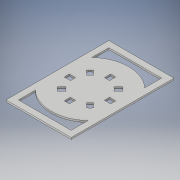
# Autodesk Inventor part: Cuerpo - Base
Saved by Autodesk Inventor 2019 (Build 230136000, 136)
## iProperties
Created: 2020-02-15
Part Number: Cuerpo - Base
Material: Genérico
Document SubType Name: Modeling
Designer: Mafer1
Density: 1 g/cm^3
Appearance: Valor por defecto
Mass: 62.4881 g
Surface Area: 432.904 cm^2
Volume: 62.4881 cm^3
ancho_base: 120.000 mm
largo_base: 200.000 mm
Author: Mafer1
Autodesk Inventor part; units mm, degrees
ref_plane "YZ Plane" through (0, 0, 0) normal (1, 0, 0) x (0, 1, 0)
ref_plane "XZ Plane" through (0, 0, 0) normal (0, 1, 0) x (-1, 0, 0)
ref_plane "XY Plane" through (0, 0, 0) normal (0, 0, 1) x (1, 0, 0)
sketch "Boceto1" plane through (0, 0, 0) normal (0, 1, 0) x (-1, 0, 0)
  line L0 (0, 0) -> (126.6, 0)
  line L1 (126.6, 0) -> (126.6, -200)
  line L2 (126.6, -200) -> (0, -200)
  line L3 (0, -200) -> (0, 0)
  dimension "d0" = 200
  dimension "d1" = 126.6
  constraints: 8 end point, 2 parallel, 1 horizontal, 1 perpendicular
  measures "d0" distance of L0.end L1.end
  measures "d1" distance between parallel lines of L3 L1
extrude "Extrusión1" add sketch "Boceto1" along normal blind 3.3
sketch "Boceto2" plane through (0, 3.3, 0) normal (0, 1, 0) x (1, 0, 0)
  circle A0 centre (-63.3, 100) radius 33.3 construction
  circle A1 centre (-63.3, 100) radius 45.3 construction
  line L0 (-114.6, 155.1217) -> (-114.6, 188)
  line L1 (-114.6, 188) -> (-12, 188)
  line L2 (-12, 188) -> (-12, 155.1217)
  line L3 (-114.6, 44.8783) -> (-114.6, 12)
  line L4 (-114.6, 12) -> (-12, 12)
  line L5 (-12, 12) -> (-12, 44.8783)
  arc A2 (-12, 155.1217) -> (-114.6, 155.1217) centre (-63.3, 100) ccw
  arc A3 (-114.6, 44.8783) -> (-12, 44.8783) centre (-63.3, 100) ccw
  line L6 (-126.6, 0) -> (0, 0) projected
  line L7 (0, 0) -> (0, 200) projected
  line L8 (0, 200) -> (-126.6, 200) projected
  line L9 (-126.6, 200) -> (-126.6, 0) projected
  line L10 (0, 200) -> (-126.6, 200) projected
  line L11 (-68.3, 54.9768) -> (-68.3, 67.0775)
  line L12 (-58.3, 54.9768) -> (-58.3, 67.0775)
  arc A4 (-68.3, 67.0775) -> (-58.3, 67.0775) centre (-63.3, 100) ccw
  arc A5 (-68.3, 54.9768) -> (-58.3, 54.9768) centre (-63.3, 100) ccw
  line L13 (-27.9282, 71.6993) -> (-36.4848, 80.2558)
  arc A6 (-34.9993, 64.6282) -> (-27.9282, 71.6993) centre (-63.3, 100) ccw
  line L14 (-34.9993, 64.6282) -> (-43.5558, 73.1848)
  arc A7 (-43.5558, 73.1848) -> (-36.4848, 80.2558) centre (-63.3, 100) ccw
  line L15 (-18.2768, 105) -> (-30.3775, 105)
  arc A8 (-18.2768, 95) -> (-18.2768, 105) centre (-63.3, 100) ccw
  line L16 (-18.2768, 95) -> (-30.3775, 95)
  arc A9 (-30.3775, 95) -> (-30.3775, 105) centre (-63.3, 100) ccw
  line L17 (-34.9993, 135.3718) -> (-43.5558, 126.8152)
  arc A10 (-27.9282, 128.3007) -> (-34.9993, 135.3718) centre (-63.3, 100) ccw
  line L18 (-27.9282, 128.3007) -> (-36.4848, 119.7442)
  arc A11 (-36.4848, 119.7442) -> (-43.5558, 126.8152) centre (-63.3, 100) ccw
  line L19 (-68.3, 145.0232) -> (-68.3, 132.9225)
  arc A12 (-58.3, 145.0232) -> (-68.3, 145.0232) centre (-63.3, 100) ccw
  line L20 (-58.3, 145.0232) -> (-58.3, 132.9225)
  arc A13 (-58.3, 132.9225) -> (-68.3, 132.9225) centre (-63.3, 100) ccw
  line L21 (-98.6718, 128.3007) -> (-90.1152, 119.7442)
  arc A14 (-91.6007, 135.3718) -> (-98.6718, 128.3007) centre (-63.3, 100) ccw
  line L22 (-91.6007, 135.3718) -> (-83.0442, 126.8152)
  arc A15 (-83.0442, 126.8152) -> (-90.1152, 119.7442) centre (-63.3, 100) ccw
  line L23 (-108.3232, 95) -> (-96.2225, 95)
  arc A16 (-108.3232, 105) -> (-108.3232, 95) centre (-63.3, 100) ccw
  line L24 (-108.3232, 105) -> (-96.2225, 105)
  arc A17 (-96.2225, 105) -> (-96.2225, 95) centre (-63.3, 100) ccw
  line L25 (-91.6007, 64.6282) -> (-83.0442, 73.1848)
  arc A18 (-98.6718, 71.6993) -> (-91.6007, 64.6282) centre (-63.3, 100) ccw
  line L26 (-98.6718, 71.6993) -> (-90.1152, 80.2558)
  arc A19 (-90.1152, 80.2558) -> (-83.0442, 73.1848) centre (-63.3, 100) ccw
  line L27 (-126.6, 200) -> (-126.6, 0) projected
  line L28 (0, 0) -> (0, 200) projected
  point P0 (-63.3, 200)
  point P1 (-126.6, 100)
  point P2 (-63.3, 200)
  point P3 (-63.3, 66.7)
  point P4 (-39.7533, 76.4533)
  point P5 (-30, 100)
  point P6 (-39.7533, 123.5467)
  point P7 (-63.3, 133.3)
  point P8 (-86.8467, 123.5467)
  point P9 (-96.6, 100)
  point P10 (-86.8467, 76.4533)
  dimension "d4" = 12
  dimension "d5" = 12
  dimension "d6" = 12
  dimension "d7" = 12
  dimension "d8" = 30
  dimension "d9" = 30
  dimension "d10" = 12
  dimension "d11" = 10
  dimension "d14" = 360
  dimension "d19" = 30
  constraints: 44 end point, 41 point on circle, 20 centre point, 4 concentric, 4 perpendicular, 3 midpoint, 3 parallel, 3 vertical, 3 vertical alignment, 2 point on line, 1 coincident, 1 collinear, 1 horizontal alignment, 89 other
  measures "d4" distance between parallel lines of L8 L1
  measures "d5" distance between parallel lines of L9 L0
  measures "d6" distance between parallel lines of L7 L2
  measures "d7" distance between parallel lines of L6 L4
  measures "d8" radial gap between concentric circles of A3 A1
  measures "d9" radial gap between concentric circles of A1 A2
  measures "d10" radial gap between concentric circles of A1 A0
  measures "d11" distance between parallel lines of L12 L11
  measures "d19" distance of point (-126.6, 100) point (-96.6, 100)
extrude "Extrusión2" cut sketch "Boceto2" against normal blind 10 contours L0 L1 L2 A2 | A3 L5 L4 L3 | L11 A4 L12 A5 | A6 L14 A7 L13 | A8 L16 A9 L15 | A10 L18 A11 L17 | A12 L20 A13 L19 | A14 L22 A15 L21 | A16 L24 A17 L23 | A18 L26 A19 L25
equation "\"d0\" = largo_base"
equation "\"d5\" = d4"
equation "\"d6\" = d4"
equation "\"d7\" = d4"
equation "\"d9\" = d8"
equation "\"d10\" = d4"
equation "\"d11\" = 0.333333 * d19"
equation "\"d19\" = d8"
equation "\"ancho_base\" = 120"
equation "\"largo_base\" = 200"
